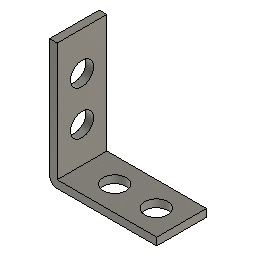
L bracket v12 (Autodesk Fusion 360 design; units mm, degrees)
Autodesk Fusion 360 part; units mm, degrees
sketch "Sketch1" plane through (0, 0, 0) normal (0, 0, 1) x (1, 0, 0)
  line L0 (0, 0) -> (89.0778, 0)
  line L1 (89.0778, 0) -> (89.0778, 41.3004)
  line L2 (89.0778, 41.3004) -> (0, 41.3004)
  line L3 (0, 41.3004) -> (0, 0)
  line L4 (0, 41.3004) -> (6.35, 41.3004)
  line L5 (6.35, 41.3004) -> (6.35, 0)
  line L6 (6.35, 0) -> (0, 0)
  line L7 (0, 0) -> (0, 41.3004)
  circle A0 centre (33.4171, 20.6502) radius 9.525
  circle A1 centre (68.046, 20.6502) radius 9.525
  point P0 (50.7316, 20.6502)
  dimension "d1" = 89.0778
  dimension "d2" = 41.3004
  dimension "d7" = 6.35
  dimension "d12" = 19.05
  dimension "d19" = 17.3145
  dimension "d20" = 17.3145
  constraint horizontal L0
  constraint vertical L1
  constraint horizontal L2
  constraint vertical L3
  constraint coincident L0.start L3.end
  constraint horizontal L4
  constraint vertical L5
  constraint horizontal L6
  constraint vertical L7
  constraint coincident L0 L5.end
  constraint equal A0 A1
  measures "d1" distance of L0.start L0.end
  measures "d2" distance of L0.start L2.end
  measures "d7" distance of L2.end L4.end
  measures "d12" diameter of A1
  measures "d19" distance of A0.centre P0
  measures "d20" distance of A1.centre P0
extrude "Extrude1" add sketch "Sketch1" along normal blind 6.35 contours L0 L2 L3 L4 L5 L6 L7 | L0 L1 L2 L5 | A0 | A1
extrude "Extrude2" add sketch "Sketch1" along normal blind 104.648 contours L0 L2 L3 L4 L5 L6 L7
fillet "Fillet1" radius 6.35 1 edges at (0, 20.6502, 0)
extrude "Extrude3" cut sketch "Sketch1" along normal blind 129.54 contours A0 | A1
sketch "Sketch2" plane through (0, 0, 0) normal (-1, 0, 0) x (0, -1, 0)
  line L0 (-41.3004, 6.35) -> (0, 6.35)
  line L1 (0, 6.35) -> (0, 104.648)
  line L2 (0, 104.648) -> (-41.3004, 104.648)
  line L3 (-41.3004, 104.648) -> (-41.3004, 6.35)
  line L4 (-20.6502, 104.648) -> (-20.6502, 6.35) construction
  circle A0 centre (-20.6502, 72.4894) radius 9.525
  circle A1 centre (-20.6502, 35.7876) radius 9.525
  dimension "d15" = 19.05
  dimension "d16" = 19.05
  constraint midpoint L2 L4.start
  constraint midpoint L0 L4.end
  constraint coincident L4 A0.centre
  constraint coincident L4 A1.centre
  measures "d15" diameter of A0
  measures "d16" diameter of A1
extrude "Extrude4" cut sketch "Sketch2" against normal blind 182.88 contours A0 | A1
equation "d20 = d19"
